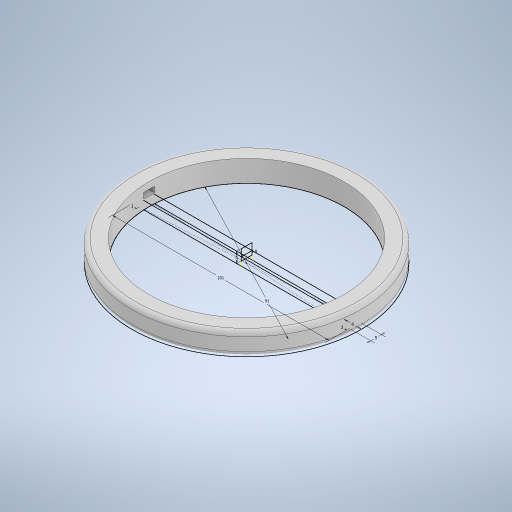
# Autodesk Inventor part: IR센서테스트
Saved by Autodesk Inventor 2023 (Build 270158000, 158)
## iProperties
Created: 2023-09-20
Part Number: IR센서테스트
Material: 일반
Document SubType Name: Modeling
Designer: rlatk
Density: 1 g/cm^3
Appearance: 기본값
Author: rlatk
Autodesk Inventor part; units mm, degrees
ref_plane "YZ Plane" through (0, 0, 0) normal (1, 0, 0) x (0, 1, 0)
ref_plane "XZ Plane" through (0, 0, 0) normal (0, 1, 0) x (-1, 0, 0)
ref_plane "XY Plane" through (0, 0, 0) normal (0, 0, 1) x (1, 0, 0)
sketch "스케치1" plane through (0, 0, 0) normal (0, 1, 0) x (-1, 0, 0)
  circle A0 centre (0, 0) radius 45.5
  circle A1 centre (0, 0) radius 53.5
  line L0 (50.5, -2.5) -> (-50.5, -2.5)
  line L1 (-50.5, -2.5) -> (-50.5, 2.5)
  line L2 (-50.5, 2.5) -> (50.5, 2.5)
  line L3 (50.5, 2.5) -> (50.5, -2.5)
  line L4 (50.5, -2.5) -> (-50.5, 2.5) construction
  line L5 (-50.5, -2.5) -> (50.5, 2.5) construction
  line L6 (-47.5, 2.5) -> (-47.5, -2.5)
  line L7 (47.5, 2.5) -> (47.5, -2.5)
  dimension "d0" = 91
  dimension "d1" = 8
  dimension "d5" = 101
  dimension "d6" = 5
  dimension "d7" = 3
  dimension "d8" = 3
  constraints: 16 end point, 4 point on line, 3 perpendicular, 2 centre point, 2 midpoint, 2 parallel, 1 coincident, 1 horizontal
  measures "d0" diameter of A0
  measures "d1" radial gap between concentric circles of A0 A1
  measures "d5" distance of L1.end L2.end
  measures "d6" distance of L0.end L1.end
  measures "d7" distance between parallel lines of L6 L1
  measures "d8" distance between parallel lines of L3 L7
extrude "돌출1" add sketch "스케치1" along normal blind 10 contours A0 L2 L7 L0 | A0 L0 L6 L2 | L2 L3 L0 L7 | L6 L0 L1 L2 | A1
fillet "모깎기1" radius 2 2 edges at (53.5, 10, 0) (53.5, 0, 0)
extrude "돌출2" cut sketch "스케치1" along normal blind 7 contours L2 L3 L0 L7 | L6 L0 L1 L2
sketch "스케치2" plane through (0, 0, 0) normal (1, 0, 0) x (0, 1, 0)
  line L0 (0, -2.5) -> (7, -2.5) projected
  line L1 (0, 2.5) -> (7, 2.5) projected
  line L2 (7, 2.5) -> (7, -2.5) projected
  line L3 (7, -2.5) -> (2, -2.5)
  line L4 (2, -2.5) -> (2, 2.5)
  line L5 (2, 2.5) -> (7, 2.5)
  line L6 (7, 2.5) -> (7, -2.5)
  line L7 (2, 2.5) -> (3.8, 2.5)
  line L8 (3.8, 2.5) -> (3.8, -2.5)
  line L9 (3.8, -2.5) -> (2, -2.5)
  line L10 (2, -2.5) -> (2, 2.5)
  point P0 (0, 0)
  point P1 (3.8, -2.5)
  dimension "d11" = 5
  dimension "d16" = 1.8
  constraints: 16 end point, 4 parallel, 2 horizontal, 2 perpendicular, 2 point on line
  measures "d11" distance of L4.end L5.end
  measures "d16" distance of L8.end L9.end
extrude "돌출3" cut sketch "스케치2" along normal blind 52.5 and the other way blind 52.5
extrude "돌출4" add sketch "스케치2" along normal blind 49 and the other way blind 49 contours L4 L1 L8 L0
sketch "스케치3" plane through (-45.4313, 3.8, -2.5) normal (0, 1, 0) x (1, 0, 0)
  line L0 (94.4313, -5) -> (94.4313, 0) projected
  line L1 (-3.5687, 0) -> (-3.5687, -5) projected
  line L2 (94.4313, -5) -> (-3.5687, -5)
  line L3 (-3.5687, -5) -> (-3.5687, 0)
  line L4 (-3.5687, 0) -> (94.4313, 0)
  line L5 (94.4313, 0) -> (94.4313, -5)
  point P0 (45.4313, -2.5)
  point P1 (-3.5687, -5)
  constraints: 8 end point, 2 parallel, 1 horizontal, 1 perpendicular
extrude "돌출5" add sketch "스케치3" along normal blind 0.5
extrude "돌출6" cut sketch "스케치3" against normal blind 1.8
extrude "돌출7" cut sketch "스케치1" along normal blind 10 contours A0 L0 L2 | L2 A0 | A0 L0
sketch "스케치4" plane through (-45.4313, 2, -2.5) normal (0, 1, 0) x (1, 0, 0)
  line L0 (-5.0687, 0) -> (95.9313, 0) projected
  line L1 (95.9313, -5) -> (-5.0687, -5) projected
  line L2 (-5.0687, -5) -> (-2.0687, -5) projected
  circle A0 centre (45.4313, -2.5) radius 45.5 projected
  line L3 (-2.0687, -5) -> (0, -5)
  line L4 (0, 0) -> (-2.0687, 0)
  line L5 (-2.0687, 0) -> (-2.0687, -5)
  circle A1 centre (45.4313, -2.5) radius 45.5
  line L6 (45.4313, -5) -> (45.4313, 0)
  line L7 (95.9313, 0) -> (-5.0687, 0)
  line L8 (-5.0687, -5) -> (95.9313, -5)
  circle A2 centre (45.4313, -2.5) radius 45.5
  line L9 (92.9313, 0) -> (92.9313, -5)
  point P0 (92.9313, -5)
  point P1 (92.9313, 0)
  point P2 (90.8625, 0)
  point P3 (90.8625, -5)
  point P4 (-2.0687, 0)
  point P5 (0, -5)
  constraints: 14 end point, 6 symmetric about line, 2 centre point, 2 midpoint, 1 coincident, 1 horizontal, 1 line through centre, 1 parallel, 1 point on line, 3 other
extrude "돌출8" add sketch "스케치4" along normal blind 1.8 contours L0 A0 L1 L5 | L0 L9 L1 A0
